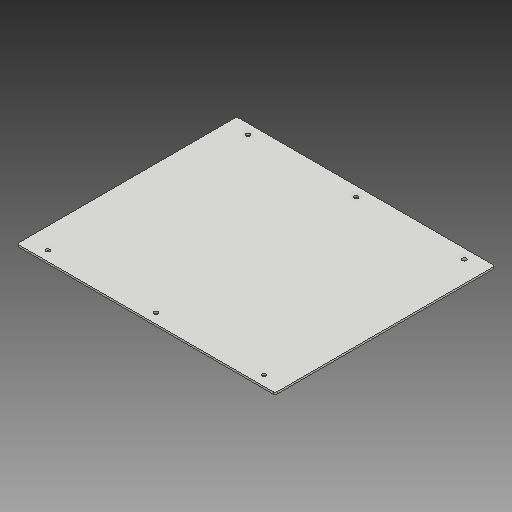
# Autodesk Inventor part: Deckel
Saved by Autodesk Inventor 2018 (Build 220112000, 112)
## iProperties
Created: 2017-11-12
Part Number: Deckel
Material: Generisch
Document SubType Name: Blech
Density: 1 g/cm^3
Sheet Metal Rule: Standard_mm
Appearance: Vorgabe
Flat Pattern Width: 22.4 cm
Flat Pattern Length: 26.3 cm
Flat Pattern Area: 589.12 cm^2
Sheet Metal Width: 224,000 mm
Sheet Metal Length: 263,000 mm
Sheet Metal Area: 58912,000 mm^2
Autodesk Inventor part; units mm, degrees
ref_plane "YZ Plane" through (0, 0, 0) normal (1, 0, 0) x (0, 1, 0)
ref_plane "XZ Plane" through (0, 0, 0) normal (0, 1, 0) x (-1, 0, 0)
ref_plane "XY Plane" through (0, 0, 0) normal (0, 0, 1) x (1, 0, 0)
sketch "Skizze1" plane through (0, 0, 0) normal (0, 0, 1) x (1, 0, 0)
  line L0 (-131.5, -112) -> (131.5, -112)
  line L1 (131.5, -112) -> (131.5, 112)
  line L2 (131.5, 112) -> (-131.5, 112)
  line L3 (-131.5, 112) -> (-131.5, -112)
  line L4 (-131.5, -112) -> (131.5, 112) construction
  line L5 (131.5, -112) -> (-131.5, 112) construction
  circle A0 centre (0, 102) radius 2.15
  line L6 (0, 156.8) -> (0, -156.8)
  circle A1 centre (-110, 102) radius 2.15
  circle A2 centre (110, 102) radius 2.15
  line L7 (-131.5, 0) -> (131.5, 0) construction
  circle A3 centre (0, -102) radius 2.15
  circle A4 centre (-110, -102) radius 2.15
  circle A5 centre (110, -102) radius 2.15
  point P0 (0, 0)
  dimension "d0" = 263
  dimension "d1" = 224
  dimension "d2" = 4.3
  dimension "d3" = 0
  dimension "d4" = 10
  dimension "d5" = 4.3
  dimension "d6" = 4.3
  dimension "d7" = 10
  dimension "d8" = 10
  dimension "d9" = 110
  dimension "d10" = 110
  measures "d0" distance of L2.end L1.end
  measures "d1" distance of L1.end L0.end
  measures "d2" diameter of A0
  measures "d3" distance from line of L6 A0.centre
  measures "d4" distance from line of L2 A0.centre
  measures "d5" diameter of A1
  measures "d6" diameter of A2
  measures "d7" distance from line of L2 A2.centre
  measures "d8" distance from line of L2 A1.centre
  measures "d9" distance of A0.centre A1.centre
  measures "d10" distance of A0.centre A2.centre
extrude "Grobblech1" add sketch "Skizze1" along normal blind 2 contours L3 L2 L6 A0 A3 L0 | L6 A3 A0 L2 L1 L0
fillet "Rundung1" radius 2 4 edges at (131.5, 112, 1) (131.5, -112, 1) (-131.5, -112, 1) (-131.5, 112, 1)
equation "\"d5\" = d2"
equation "\"d6\" = d2"
equation "\"d7\" = d4"
equation "\"d8\" = d4"
equation "\"d11\" = Stärke"
equation "\"Biegeradius\" = Stärke"
equation "\"BreiteBiegungsfreistellung\" = Stärke"
equation "\"TiefeBiegungsfreistellung\" = 0.5 * Stärke"
equation "\"GrößeEckenfreistellung\" = 4 * Stärke"
equation "\"MinimalRest\" = 2 * Stärke"
equation "\"Übergangsradius\" = Biegeradius"
equation "\"JacobiRadiusGröße\" = Biegeradius"
equation "\"Abstandsgröße\" = Stärke"
equation "\"Stärke\" = 2"
